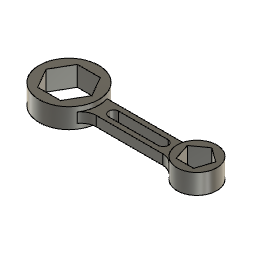
Exercise_2 (Autodesk Fusion 360 design; units mm, degrees)
Autodesk Fusion 360 part; units mm, degrees
note: some values were not read from the file. Chosen so that the rebuilt part matches the saved one: which face or edge a step refers to.
sketch "Sketch1" plane through (0, 0, 0) normal (0, 0, 1) x (1, 0, 0)
  circle A0 centre (0, 0) radius 30
  circle A1 centre (129, 0) radius 20
  line L0 (28.2843, 10) -> (111.6795, 10)
  line L1 (28.2843, -10) -> (111.6795, -10)
  line L2 (44.9819, -5) -> (94.9819, -5)
  line L3 (44.9819, 5) -> (94.9819, 5)
  arc A2 (44.9819, 5) -> (44.9819, -5) centre (44.9819, 0) ccw
  arc A3 (94.9819, -5) -> (94.9819, 5) centre (94.9819, 0) ccw
  dimension "d1" = 60
  dimension "d2" = 40
  dimension "d3" = 129
  dimension "d4" = 10
  dimension "d5" = 20
  constraint coincident A0.centre origin
  constraint coincident A0 L0.start
  constraint coincident A1 L0.end
  constraint horizontal L0
  constraint tangent L3 A3
  constraint tangent L3 A2
  constraint parallel L0 L3
  constraint parallel L0 L2
  measures "d1" diameter of A0
  measures "d2" diameter of A1
  measures "d3" distance of A0.centre A1.centre
  measures "d4" distance of A0.centre L0
extrude "Extrude1" add sketch "Sketch1" along normal mid plane 20 contours A0 | A1 makes body 1 at (148.9006, -1.9914, -3.3333) makes body 2 at (6.6746, 11.603, 10)
extrude "Extrude2" add sketch "Sketch1" along normal mid plane 10 contours A0 A1 L0 L1 bodies 1 2
sketch "Sketch2" plane through (0, 0, 10) normal (0, 0, 1) x (-1, 0, 0)
  circle A0 centre (0, 0) radius 30
  line L0 (11.547, -20) -> (23.094, 0)
  line L1 (23.094, 0) -> (11.547, 20)
  line L2 (11.547, 20) -> (-11.547, 20)
  line L3 (-11.547, 20) -> (-23.094, 0)
  line L4 (-23.094, 0) -> (-11.547, -20)
  line L5 (-11.547, -20) -> (11.547, -20)
  dimension "d14" = 20
  constraint coincident A0.centre origin
  measures "d14" distance of A0.centre L5
extrude "Extrude3" cut sketch "Sketch2" against normal up to surface (20 mm away) contours L0 L1 L2 L3 L4 L5 bodies 1
sketch "Sketch3" plane through (0, 0, 10) normal (0, 0, 1) x (-1, 0, 0)
  circle A0 centre (-129, 0) radius 20
  line L0 (-129, -15) -> (-114.7342, -4.6353)
  line L1 (-114.7342, -4.6353) -> (-120.1832, 12.1353)
  line L2 (-120.1832, 12.1353) -> (-137.8168, 12.1353)
  line L3 (-137.8168, 12.1353) -> (-143.2658, -4.6353)
  line L4 (-143.2658, -4.6353) -> (-129, -15)
  point P0 (-129, 0)
  dimension "d17" = 15
  constraint coincident P0 A0.centre
  measures "d17" distance of L0.start P0
extrude "Extrude4" cut sketch "Sketch3" against normal up to surface (20 mm away) contours L0 L1 L2 L3 L4 bodies 1
fillet "Fillet1" radius 15 1 edges at (111.6795, -10, 0) on bodies 1
fillet "Fillet2" radius 15 1 edges at (28.2843, -10, 0) on bodies 1
